Autodesk Inventor part; units mm, degrees
(part 2 of 2)
extrude "Выдавливание14" cut sketch "Эскиз15" against normal blind 1
sketch "Эскиз16" plane through (-0.6771, -3.1253, 47.8094) normal (0.9999978, 0, 0.0021195) x (0.0021195, 0, -0.9999978)
  line L0 (0, 0) -> (0, 14.0669) projected
  line L1 (23.5386, 0) -> (0, 0) projected
  line L2 (7.7784, 0) -> (0, 14.0669)
  point P0 (47.8108, 3.1253)
  constraints: 2 end point, 1 other
ref_plane "РабПлоскость6" through (-20.0626, 1.6111, 45.5891) normal (0.5, 0, 0.8660254) x (0.8660254, 0, -0.5)
extrude "Выдавливание15" add sketch "Эскиз16" against normal up to surface surface through (-20.0626, 1.6111, 45.5891) normal (0.5, 0, 0.8660254)
sketch "Эскиз17" plane through (-66.4, -10, 11.3065) normal (-0.9999978, 0, -0.0021195) x (-0.0021195, 0, 0.9999978)
  line L0 (36.3635, 20.9416) -> (36.3635, 6.8747) projected
  line L1 (0, 6.8747) -> (36.3635, 6.8747) projected
  line L2 (28.6929, 6.8747) -> (36.3635, 20.9416)
  point P0 (-11.4473, 10)
  constraints: 2 end point, 1 other
ref_plane "РабПлоскость7" through (-56.7244, -3.388, 39.9684) normal (-0.5, 0, 0.8660254) x (0.8660254, 0, 0.5)
extrude "Выдавливание16" add sketch "Эскиз17" along normal up to surface surface through (-56.7244, -3.388, 39.9684) normal (-0.5, 0, 0.8660254)
chamfer "Фаска1" distance 4 angle 45 1 edges at (-33.5792, -2.237, 48.7377)
ref_plane "РабПлоскость8" through (-33.518, -3.1253, 23.8341) normal (0, -1, 0) x (0.9999978, 0, 0.0021189)
sketch "Эскиз18" plane through (-33.518, -3.1253, 23.8341) normal (0, -1, 0) x (0.9999978, 0, 0.0021189)
  line L0 (-26.4158, -15.8106) -> (-19.6239, -19.7512) projected
  line L1 (-19.6239, -19.7512) -> (-11.5461, -15.1102) projected
  line L2 (-11.5461, -15.1102) -> (-8.082, -15.1176) projected
  line L3 (-8.082, -15.1176) -> (-0.024, -19.7927) projected
  line L4 (-0.024, -19.7927) -> (8.0538, -15.1518) projected
  line L5 (8.0538, -15.1518) -> (11.5179, -15.1591) projected
  line L6 (11.5179, -15.1591) -> (19.576, -19.8342) projected
  line L7 (19.576, -19.8342) -> (26.3845, -15.9225) projected
  arc A0 (26.3845, -15.9225) -> (29.3884, -13.9991) centre (28.4843, -15.8945) ccw projected
  line L8 (29.3884, -13.9991) -> (29.4126, -2.5649) projected
  line L9 (29.4126, -2.5649) -> (29.4119, -2.5649) projected
  line L10 (29.4119, -2.5649) -> (29.4119, -1.8793) projected
  line L11 (29.4119, -1.8793) -> (28.664, -1.8793) projected
  line L12 (28.664, -1.8793) -> (27.682, -1.8773) projected
  line L13 (27.682, -1.8773) -> (19.6239, 2.7979) projected
  line L14 (19.6239, 2.7979) -> (19.6486, 14.43) projected
  line L15 (19.6486, 14.43) -> (19.6205, 14.43) projected
  line L16 (19.6205, 14.43) -> (19.6205, 15.1155) projected
  line L17 (19.6205, 15.1155) -> (18.9, 15.1155) projected
  line L18 (18.9, 15.1155) -> (17.918, 15.1176) projected
  line L19 (17.918, 15.1176) -> (16.1641, 16.1351) projected
  line L20 (16.1641, 16.1351) -> (16.1284, 16.1352) projected
  line L21 (16.1284, 16.1352) -> (10.5788, 19.3458) projected
  line L22 (10.5788, 19.3458) -> (10.355, 19.4756) projected
  line L23 (10.355, 19.4756) -> (10.3544, 19.4756) projected
  line L24 (10.3544, 19.4756) -> (9.8319, 19.7778) projected
  line L25 (9.8319, 19.7778) -> (9.0875, 19.3489) projected
  line L26 (9.0875, 19.3489) -> (8.8632, 19.22) projected
  line L27 (8.8632, 19.22) -> (8.8634, 19.2198) projected
  line L28 (8.8634, 19.2198) -> (8.1285, 18.7964) projected
  line L29 (8.1285, 18.7964) -> (8.1258, 18.7964) projected
  line L30 (8.1258, 18.7964) -> (1.7821, 15.1518) projected
  line L31 (1.7821, 15.1518) -> (-1.682, 15.1591) projected
  line L32 (-1.682, 15.1591) -> (-3.4025, 16.1573) projected
  line L33 (-3.4025, 16.1573) -> (-3.4381, 16.1573) projected
  line L34 (-3.4381, 16.1573) -> (-9.0212, 19.3873) projected
  line L35 (-9.0212, 19.3873) -> (-9.2449, 19.5171) projected
  line L36 (-9.2449, 19.5171) -> (-9.2456, 19.5171) projected
  line L37 (-9.2456, 19.5171) -> (-9.768, 19.8194) projected
  line L38 (-9.768, 19.8194) -> (-10.5125, 19.3904) projected
  line L39 (-10.5125, 19.3904) -> (-10.7368, 19.2616) projected
  line L40 (-10.7368, 19.2616) -> (-10.7366, 19.2613) projected
  line L41 (-10.7366, 19.2613) -> (-11.4715, 18.8379) projected
  line L42 (-11.4715, 18.8379) -> (-11.4742, 18.8379) projected
  line L43 (-11.4742, 18.8379) -> (-17.8178, 15.1933) projected
  line L44 (-17.8178, 15.1933) -> (-18.7999, 15.1954) projected
  line L45 (-18.7999, 15.1954) -> (-19.5666, 15.1954) projected
  line L46 (-19.5666, 15.1954) -> (-19.5666, 14.1737) projected
  line L47 (-19.5666, 14.1737) -> (-19.552, 14.1821) projected
  line L48 (-19.552, 14.1821) -> (-19.576, 2.8648) projected
  line L49 (-19.576, 2.8648) -> (-19.5765, 2.8651) projected
  line L50 (-19.5765, 2.8651) -> (-19.5765, 2.8806) projected
  line L51 (-19.5765, 2.8806) -> (-27.6538, -1.76) projected
  line L52 (-27.6538, -1.76) -> (-29.3858, -1.7563) projected
  line L53 (-29.3858, -1.7563) -> (-29.4115, -13.8745) projected
  arc A1 (-29.4115, -13.8745) -> (-26.4158, -15.8106) centre (-28.5155, -15.7738) ccw projected
  line L54 (-23.0824, 6.3133) -> (-23.0824, 16.235) projected
  line L55 (-23.0824, 16.235) -> (-9.7831, 23.8758) projected
  line L56 (-9.7831, 23.8758) -> (9.8168, 23.8342) projected
  line L57 (9.8168, 23.8342) -> (9.8426, 23.8193) projected
  line L58 (9.8426, 23.8193) -> (9.8685, 23.8341) projected
  line L59 (9.8685, 23.8341) -> (19.6744, 18.1449) projected
  line L60 (19.6744, 18.1449) -> (23.1486, 16.1272) projected
  line L61 (23.1486, 16.1272) -> (23.1486, 14.4226) projected
  line L62 (23.1486, 14.4226) -> (23.1314, 6.3133) projected
  line L63 (25.4773, 3.4483) -> (23.1314, 6.3133) projected
  line L64 (25.4773, 3.4483) -> (29.4384, 1.1501) projected
  line L65 (29.4384, 1.1501) -> (32.9126, -0.8676) projected
  line L66 (32.9126, -0.8676) -> (32.9126, -2.5723) projected
  line L67 (32.9126, -2.5723) -> (32.8873, -14.5204) projected
  line L68 (32.8873, -14.5204) -> (32.8873, -16.2251) projected
  line L69 (32.8873, -16.2251) -> (29.3974, -18.2281) projected
  line L70 (29.3974, -18.2281) -> (19.5674, -23.8757) projected
  line L71 (19.5674, -23.8757) -> (9.7794, -18.1969) projected
  line L72 (9.7794, -18.1969) -> (3.4538, -21.8311) projected
  line L73 (3.4538, -21.8311) -> (0.0176, -23.8308) projected
  line L74 (0.0176, -23.8308) -> (-9.8165, -18.153) projected
  line L75 (-9.8165, -18.153) -> (-19.6325, -23.7926) projected
  line L76 (-19.6325, -23.7926) -> (-29.4384, -18.1034) projected
  line L77 (-29.4384, -18.1034) -> (-32.9126, -16.0857) projected
  line L78 (-32.9126, -16.0857) -> (-32.9126, -14.381) projected
  line L79 (-32.9126, -14.381) -> (-32.8873, -2.4329) projected
  line L80 (-32.8873, -2.4329) -> (-32.8873, -0.7282) projected
  line L81 (-32.8873, -0.7282) -> (-29.3974, 1.2748) projected
  line L82 (-29.3974, 1.2748) -> (-25.6142, 3.4483) projected
  line L83 (-23.0824, 6.3133) -> (-25.6142, 3.4483) projected
  point P0 (33.4674, -23.9051)
extrude "Выдавливание17" cut sketch "Эскиз18" against normal blind 10 contours A1 L53 L52 L51 L48 L47 L46 L45 L44 L43 L42 L41 L39 L38 L37 L35 L34 L33 L32 L31 L30 L29 L28 L26 L25 L24 L22 L21 L20 L19 L18 L17 L16 L15 L14 L13 L12 L11 L10 L8 A0 L7 L6 L5 L4 L3 L2 L1 L0
sketch "Эскиз19" plane through (-58.009, 6.8113, 2.8342) normal (0, 1, 0) x (1, 0, 0)
  line L0 (55.609, -0.1658) -> (51.409, -0.1658) projected
  line L1 (57.41, -4.8431) -> (57.41, 2.8342) projected
  line L2 (-8.391, 2.8342) -> (57.41, 2.8342) projected
  line L3 (-8.391, 2.8342) -> (-8.391, -4.8446) projected
  line L4 (0, 0) -> (-8.391, -4.8446) projected
  line L5 (0, 0) -> (9.8179, 0) projected
  line L6 (14.713, -2.8262) -> (9.8179, 0) projected
  line L7 (19.6321, 0) -> (14.713, -2.8262) projected
  line L8 (19.6321, 0) -> (29.4179, 0) projected
  line L9 (34.309, -2.8238) -> (29.4179, 0) projected
  line L10 (39.2, 0) -> (34.309, -2.8238) projected
  line L11 (39.2, 0) -> (49.0179, 0) projected
  line L12 (53.9269, -2.8342) -> (49.0179, 0) projected
  line L13 (57.41, -4.8431) -> (53.9269, -2.8342) projected
  point P0 (58.009, 2.8342)
ref_plane "РабПлоскость9" through (-66.4132, 5.4, -3.8306) normal (0, -1, 0) x (1, 0, 0)
extrude "Выдавливание18" cut sketch "Эскиз19" against normal up to surface (1.4113 mm away)
sketch "Эскиз20" plane through (-66.4, 5.4, 0) normal (0, 1, 0) x (1, 0, 0)
  point P0 (66.4, 0)
sketch "Эскиз21" plane through (-66.4, 5.4, 0) normal (0, 1, 0) x (1, 0, 0)
  line L0 (62.767, -3) -> (62.767, -2.8342) projected
  line L1 (61.0331, -3) -> (62.767, -3) projected
  line L2 (61.0331, -2.8342) -> (61.0331, -3) projected
  line L3 (62.767, -2.8342) -> (61.0331, -2.8342) projected
  line L4 (3.033, -3) -> (4.7669, -3) projected
  line L5 (3.033, -2.8342) -> (3.033, -3) projected
  line L6 (4.7669, -2.8342) -> (3.033, -2.8342) projected
  line L7 (4.7669, -3) -> (4.7669, -2.8342) projected
  line L8 (0, 0) -> (65.8011, 0) projected
  line L9 (0, -7.6788) -> (0, 0) projected
  line L10 (8.391, -2.8342) -> (0, -7.6788) projected
  line L11 (18.209, -2.8342) -> (8.391, -2.8342) projected
  line L12 (23.104, -5.6604) -> (18.209, -2.8342) projected
  line L13 (28.0231, -2.8342) -> (23.104, -5.6604) projected
  line L14 (37.809, -2.8342) -> (28.0231, -2.8342) projected
  line L15 (42.7, -5.658) -> (37.809, -2.8342) projected
  line L16 (47.591, -2.8342) -> (42.7, -5.658) projected
  line L17 (57.409, -2.8342) -> (47.591, -2.8342) projected
  line L18 (62.3179, -5.6684) -> (57.409, -2.8342) projected
  line L19 (65.8011, -7.6773) -> (62.3179, -5.6684) projected
  line L20 (65.8011, 0) -> (65.8011, -7.6773) projected
  line L21 (67, -1.8301) -> (0, -1.8301) projected
  point P0 (66.4, 0)
  point P1 (65.8011, -1.8301)
extrude "Выдавливание19" add sketch "Эскиз21" along normal blind 10 contours L1 L2 L3 L0 | L5 L6 L7 L4 | L21 L20 L19 L18 L17 L16 L15 L14 L13 L12 L11 L10 L9
sketch "Эскиз22" plane through (-0.5989, 5.4, 1.8301) normal (0, 0, -1) x (-1, 0, 0)
  circle A0 centre (61.3011, 3.4873) radius 2.1 projected
  line L0 (65.8011, 0) -> (0, 0) projected
  line L1 (65.8011, 0) -> (65.8011, 10) projected
  line L2 (0, 10) -> (65.8011, 10) projected
  line L3 (0, 0) -> (0, 10) projected
  circle A1 centre (3.301, 3.4873) radius 2.1 projected
  point P0 (-0.5989, -5.4)
extrude "Выдавливание20" cut sketch "Эскиз22" against normal blind 10 contours A0 | A1
sketch "Эскиз23" plane through (-0.5989, 5.4, 1.8301) normal (0, 0, -1) x (-1, 0, 0)
  circle A0 centre (3.301, 3.4873) radius 2.1 projected
  circle A1 centre (61.3011, 3.4873) radius 2.1 projected
  line L0 (65.8011, 0) -> (0, 0) projected
  line L1 (65.8011, 0) -> (65.8011, 10) projected
  line L2 (0, 10) -> (65.8011, 10) projected
  line L3 (0, 0) -> (0, 10) projected
  line L4 (-1.1989, 6.8118) -> (65.8011, 6.8118) projected
  line L5 (65.8011, 0) -> (0, 0) projected
  line L6 (0, 0) -> (0, -15.4) projected
  line L7 (65.8011, -15.4) -> (0, -15.4) projected
  line L8 (65.8011, -15.4) -> (65.8011, 0) projected
  line L9 (65.8011, 0) -> (0, 0) projected
  line L10 (65.8011, -15.4) -> (65.8011, 0) projected
  point P0 (-0.5989, -5.4)
  point P1 (0, 6.8118)
ref_plane "РабПлоскость10" through (-66.445, 4.957, -3.6699) normal (0, 0, -1) x (0, 1, 0)
extrude "Выдавливание21" add sketch "Эскиз23" along normal up to surface (5.4999 mm away) contours L8 L7 L6 L0 | L4 L3 L2 L1
sketch "Эскиз24" plane through (-0.6877, -10, 52.8094) normal (-0.0021195, 0, 0.9999978) x (0.9999978, 0, 0.0021195)
  line L0 (-65.8001, 7.763) -> (0, 7.763) projected
  line L1 (0, 7.763) -> (0, 20.9416) projected
  line L2 (0, 20.9416) -> (-65.8001, 20.9416) projected
  line L3 (-65.8001, 20.9416) -> (-65.8001, 7.763) projected
  circle A0 centre (-38.6915, 14.9416) radius 2 projected
  circle A1 centre (-28.0253, 14.9416) radius 2 projected
  point P0 (0.5757, 10)
extrude "Выдавливание22" cut sketch "Эскиз24" against normal blind 1.5
sketch "Эскиз25" plane through (-0.6845, -10, 51.3094) normal (-0.0021195, 0, 0.9999978) x (0.9999978, 0, 0.0021195)
  line L0 (0, 7.763) -> (-65.8001, 7.763) projected
  line L1 (-65.8001, 3.763) -> (0, 3.763) projected
  line L2 (0, 7.763) -> (0, 3.763)
  line L3 (0, 6.8747) -> (0, 20.9416) projected
  line L4 (-65.8001, 7.763) -> (-65.8001, 3.763)
  line L5 (-65.8042, 6.8747) -> (-65.8042, 0) projected
  point P0 (0.5757, 10)
  constraints: 4 end point, 1 collinear, 1 parallel
extrude "Выдавливание23" cut sketch "Эскиз25" along normal blind 1.5
equation "\"Радиус_гибки\" = Толщина"
equation "\"Ширина_просечки\" = Толщина"
equation "\"Глубина_просечки\" = 0.5 * Толщина"
equation "\"Размер_просечки\" = 4 * Толщина"
equation "\"Мин_остаток\" = 2 * Толщина"
equation "\"Радиус_перехода\" = Радиус_гибки"
equation "\"Радиус_Якоби\" = Радиус_гибки"
equation "\"Размер_зазора\" = Толщина"
equation "\"Толщина\" = 3.048"
